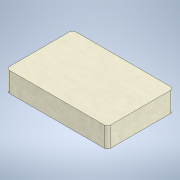
# Autodesk Inventor part: PlayerCards_All
Saved by Autodesk Inventor 2021 (Build 250183000, 183)
## iProperties
Created: 2023-03-16
Part Number: PlayerCards_All
Material: Paper
Document SubType Name: Modeling
Designer: Bradley
Density: 0.93 g/cm^3
Appearance: Cardboard - Chipboard
Author: Bradley
Autodesk Inventor part; units mm, degrees
ref_plane "YZ Plane" through (0, 0, 0) normal (1, 0, 0) x (0, 1, 0)
ref_plane "XZ Plane" through (0, 0, 0) normal (0, 1, 0) x (-1, 0, 0)
ref_plane "XY Plane" through (0, 0, 0) normal (0, 0, 1) x (1, 0, 0)
sketch "Sketch1" plane through (0, 0, 0) normal (0, 1, 0) x (-1, 0, 0)
  line L0 (30, 21) -> (-30, 21)
  line L1 (-32, 19) -> (-32, -19)
  line L2 (-30, -21) -> (30, -21)
  line L3 (32, -19) -> (32, 19)
  line L4 (32, 21) -> (-32, -21) construction
  line L5 (-32, 21) -> (32, -21) construction
  arc A0 (30, -21) -> (32, -19) centre (30, -19) ccw
  arc A1 (32, 19) -> (30, 21) centre (30, 19) ccw
  arc A2 (-30, 21) -> (-32, 19) centre (-30, 19) ccw
  arc A3 (-32, -19) -> (-30, -21) centre (-30, -19) ccw
  point P0 (0, 0)
  dimension "d0" = 64
  dimension "d1" = 42
  dimension "d2" = 2
  constraints: 12 end point, 8 point on circle, 8 point on line, 8 tangent, 4 centre point, 3 equal radius, 2 midpoint, 2 parallel, 1 horizontal, 1 perpendicular
  measures "d0" distance of L5.end L4.end
  measures "d1" distance of L4.end L5.start
  measures "d2" radius of A0
extrude "Extrusion1" add sketch "Sketch1" along normal mid plane 12.7
body "Solid1"
